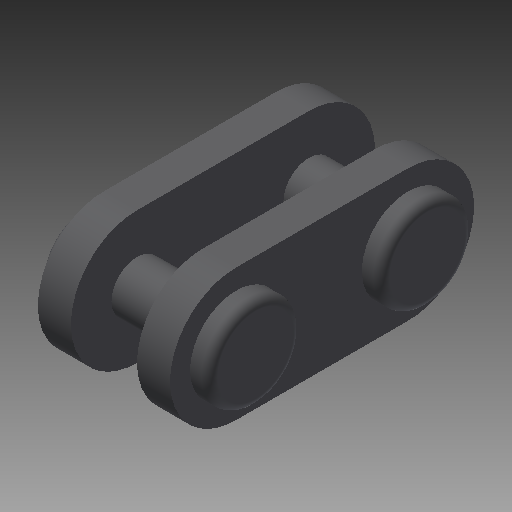
# Autodesk Inventor part: 305103-M-KOMP
Saved by Autodesk Inventor 2018 (Build 220112000, 112)
## iProperties
Category: PARTsolutions
Company: DESTACO
Created: 2018-01-28
Part Number: 305103-M-KOMP
Catalog Web Link: www.cadenas.de
Description: 305103-M-KOMP-Zwischenstuck
Vendor: DESTACO
Document SubType Name: Modeling
Designer: psAdmin
Manufacturer: DESTACO
Mass: 0.705079 g
Surface Area: 8.31862 cm^2
Volume: 0.705079 cm^3
Density: 1 g/cm^3
Material: Generic
Appearance: PSOLRGB-192-192-192
PSOL_IDENT_0: {$CADENAS_DATA\23d-libs\destaco\destaco_gmbh\man_spann\horizontalspanner\kompakt\u_kompakt_parts\zwi
PSOL_IDENT_1: schenstuck_u_komp.prj},168 {VTYP=3D},{NB=305103-M-KOMP},{LINA=305103-M-KOMP},{NN=305103-M-KOMP},{DAT
PSOL_IDENT_2: E=20.09.2016 07:53:11},{GEOMDATE=28.06.2006},{VERSION=v1},{LINEID=10},{LINESUBID=-1},{WBVAR=}  {NB=3
PSOL_IDENT_3: 05103-M-KOMP},{LINA=305103-M-KOMP},{KT=DUMMY},{MODELL=305103-M-KOMP},{SIZE=1.000}
NN: 305103-M-KOMP
NT: Zwischenstuck
NB: 305103-M-KOMP
NBSYN: $MODELL.
LINA: 305103-M-KOMP
MODELL: 305103-M-KOMP
SIZE: 1.000
SUPPLIER: DESTACO
ARTICLENO: 305103-M-KOMP
BOMINFO: 305103-M-KOMP
CREATOR: CADENAS GmbH
Title: 305103-M-KOMP
Author: Cadenas PARTsolutions
Comments: Zwischenstuck
Autodesk Inventor part; units mm, degrees
sketch "Skizze_1" plane through (0, 0, 0) normal (0, 1, 0) x (-1, 0, 0)
  line L0 (4, 14.4) -> (2, 14.4)
  line L1 (2, 14.4) -> (2, -4)
  line L2 (2, -4) -> (4, -4)
  line L3 (4, -4) -> (4, 14.4)
  constraints: 8 end point
extrude "Extrusion1" add sketch "Skizze_1" along normal mid plane 8
sketch "Skizze_2" plane through (0, 0, 0) normal (0, 1, 0) x (-1, 0, 0)
  line L0 (-5.17, 0) -> (0, 0)
  line L1 (5.17, 0) -> (5.17, -2.29)
  arc A0 (4.67, -2.79) -> (5.17, -2.29) centre (4.67, -2.29) ccw
  line L2 (4.67, -2.79) -> (4, -2.79)
  line L3 (4, -2.79) -> (4, -1.55)
  line L4 (4, -1.55) -> (-4, -1.55)
  line L5 (-4, -1.55) -> (-4, -2.79)
  line L6 (-4, -2.79) -> (-4.67, -2.79)
  arc A1 (-5.17, -2.29) -> (-4.67, -2.79) centre (-4.67, -2.29) ccw
  line L7 (-5.17, -2.29) -> (-5.17, 0)
  line L8 (-5.17, 0) -> (5.17, 0)
  constraints: 18 end point, 4 point on circle, 2 centre point
revolve "Revolution1" add sketch "Skizze_2" angle 360 about axis through (5.17, 0, 0) along (1, 0, 0)
sketch "Skizze_3" plane through (0, 0, 0) normal (0, 1, 0) x (-1, 0, 0)
  line L0 (-5.17, 10.4) -> (0, 10.4)
  line L1 (5.17, 10.4) -> (5.17, 8.11)
  arc A0 (4.67, 7.61) -> (5.17, 8.11) centre (4.67, 8.11) ccw
  line L2 (4.67, 7.61) -> (4, 7.61)
  line L3 (4, 7.61) -> (4, 8.85)
  line L4 (4, 8.85) -> (-4, 8.85)
  line L5 (-4, 8.85) -> (-4, 7.61)
  line L6 (-4, 7.61) -> (-4.67, 7.61)
  arc A1 (-5.17, 8.11) -> (-4.67, 7.61) centre (-4.67, 8.11) ccw
  line L7 (-5.17, 8.11) -> (-5.17, 10.4)
  line L8 (-5.17, 10.4) -> (5.17, 10.4)
  constraints: 18 end point, 4 point on circle, 2 centre point
revolve "Revolution2" add sketch "Skizze_3" angle 360 about axis through (5.17, 0, 10.4) along (1, 0, 0)
sketch "Skizze_4" plane through (0, 0, 0) normal (0, 1, 0) x (-1, 0, 0)
  line L0 (-2, 14.4) -> (-4, 14.4)
  line L1 (-4, 14.4) -> (-4, -4)
  line L2 (-4, -4) -> (-2, -4)
  line L3 (-2, -4) -> (-2, 14.4)
  constraints: 8 end point
extrude "Extrusion2" add sketch "Skizze_4" along normal mid plane 8
sketch "Skizze_5" plane through (0, 0, 0) normal (1, 0, 0) x (0, 1, 0)
  line L0 (-20, 30) -> (-20, -40)
  line L1 (-20, -40) -> (10, -40)
  line L2 (10, -40) -> (10, 30)
  line L3 (10, 30) -> (-20, 30)
  arc A0 (4, 10.4) -> (-4, 10.4) centre (0, 10.4) ccw
  line L4 (-4, 10.4) -> (-4, 0)
  arc A1 (-4, 0) -> (4, 0) centre (0, 0) ccw
  line L5 (4, 0) -> (4, 10.4)
  constraints: 12 end point, 4 point on circle, 2 centre point
extrude "Extrusion3" cut sketch "Skizze_5" along normal mid plane 20
ref_plane "ZS1_XY" through (0, 0, 0) normal (1, 0, 0) x (0, 0, -1)
ref_plane "ZS1_YZ" through (0, 0, 0) normal (0, 0, -1) x (0, 1, 0)
ref_plane "ZS1_ZX" through (0, 0, 0) normal (0, 1, 0) x (1, 0, 0)
ref_plane "ZS2_XY" through (0, 0, 10.4) normal (1, 0, 0) x (0, 0, -1)
ref_plane "ZS2_YZ" through (0, 0, 10.4) normal (0, 0, -1) x (0, 1, 0)
ref_plane "ZS2_ZX" through (0, 0, 10.4) normal (0, 1, 0) x (1, 0, 0)
body "Solid1"
